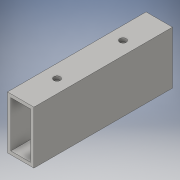
# Autodesk Inventor part: Motor Tension Block Mount
Saved by Autodesk Inventor 2016 SP2 (Build 200236200, 236)
## iProperties
Created: 2018-02-02
Part Number: Motor Tension Block Mount
Material: Generic
Document SubType Name: Modeling
Designer: CAD
Density: 1 g/cm^3
Appearance: Default
Author: CAD
Autodesk Inventor part; units mm, degrees
ref_plane "YZ Plane" through (0, 0, 0) normal (1, 0, 0) x (0, 1, 0)
ref_plane "XZ Plane" through (0, 0, 0) normal (0, 1, 0) x (-1, 0, 0)
ref_plane "XY Plane" through (0, 0, 0) normal (0, 0, 1) x (1, 0, 0)
sketch "Sketch1" plane through (0, 0, 0) normal (0, 0, 1) x (1, 0, 0)
  line L0 (-12.6521, 8.2446) -> (12.7479, 8.2446)
  line L1 (12.7479, 8.2446) -> (12.7479, -42.5554)
  line L2 (12.7479, -42.5554) -> (-12.6521, -42.5554)
  line L3 (-12.6521, -42.5554) -> (-12.6521, 8.2446)
  line L4 (9.5729, 5.0696) -> (-9.4771, 5.0696)
  line L5 (-9.4771, 5.0696) -> (-9.4771, -39.3804)
  line L6 (-9.4771, -39.3804) -> (9.5729, -39.3804)
  line L7 (9.5729, -39.3804) -> (9.5729, 5.0696)
  point P0 (0, 0)
  dimension "d1" = 25.4
  dimension "d4" = 50.8
  dimension "d5" = 3.175
  constraints: 16 end point, 2 horizontal, 2 perpendicular, 1 vertical, 3 other
  measures "d1" distance of L0.start L0.end
  measures "d4" distance of L0.end L1.end
  measures "d5" distance between parallel lines of L0 L4
extrude "Extrusion1" add sketch "Sketch1" along normal blind 133.35
sketch "Sketch2" plane through (-12.6521, 8.2446, 0) normal (0, 1, 0) x (1, 0, 0)
  line L0 (25.4, 0) -> (25.4, -133.35) projected
  line L1 (25.4, -133.35) -> (0, -133.35) projected
  point P0 (12.6521, 0)
  point P1 (12.7, -34.925)
  point P2 (12.7, -98.425)
  dimension "d8" = 63.5
  dimension "d9" = 12.7
  dimension "d10" = 12.7
  dimension "d11" = 34.925
  measures "d8" distance of point (12.7, -34.925) point (12.7, -98.425)
  measures "d9" distance from line of L0 point (12.7, -34.925)
  measures "d10" distance from line of L0 point (12.7, -98.425)
  measures "d11" distance from line of L1 point (12.7, -98.425)
hole "Hole1" at (0.0479, 8.2446, 34.925) at (0.0479, 8.2446, 98.425) direction (0, -1, 0) diameter 6.35 end through all
body "Solid1"
